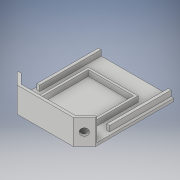
# Autodesk Inventor part: bottom-housing
Saved by Autodesk Inventor 2018 (Build 220112000, 112)
## iProperties
Created: 2019-10-14
Part Number: bottom-housing
Material: Generic
Document SubType Name: Modeling
Designer: jklei
Density: 1 g/cm^3
Appearance: Default
Author: jklei
Autodesk Inventor part; units mm, degrees
ref_plane "YZ Plane" through (0, 0, 0) normal (1, 0, 0) x (0, 1, 0)
ref_plane "XZ Plane" through (0, 0, 0) normal (0, 1, 0) x (-1, 0, 0)
ref_plane "XY Plane" through (0, 0, 0) normal (0, 0, 1) x (1, 0, 0)
sketch "Sketch1" plane through (0, 0, 0) normal (0, 1, 0) x (-1, 0, 0)
  line L0 (0, 0) -> (88.9, 0)
  line L1 (88.9, 0) -> (88.9, -101.6)
  line L2 (88.9, -101.6) -> (0, -101.6)
  line L3 (0, -101.6) -> (0, 0)
  dimension "d0" = 88.9
  dimension "d1" = 101.6
  constraints: 8 end point, 2 parallel, 1 horizontal, 1 perpendicular
  measures "d0" distance of L1.end L2.end
  measures "d1" distance of L0.end L1.end
extrude "Extrusion1" add sketch "Sketch1" along normal blind 3.175
chamfer "Chamfer1" distance 12.7 angle 45 2 edges at (-88.9, 1.5875, 0) (0, 1.5875, 0)
sketch "Sketch9" plane through (0, 3.175, 0) normal (0, 1, 0) x (1, 0, 0)
  line L0 (0, 12.7) -> (-12.7, 0) projected
  line L1 (0, 12.7) -> (0, 101.6) projected
  line L2 (0, 101.6) -> (-88.9, 101.6) projected
  line L3 (-88.9, 101.6) -> (-88.9, 12.7) projected
  line L4 (-76.2, 0) -> (-88.9, 12.7) projected
  line L5 (-76.2, 0) -> (-12.7, 0) projected
  line L6 (-3.175, 14.0151) -> (-14.0151, 3.175)
  line L7 (-14.0151, 3.175) -> (-74.8849, 3.175)
  line L8 (-74.8849, 3.175) -> (-85.725, 14.0151)
  line L9 (-88.9, 101.6) -> (0, 101.6) projected
  line L10 (-85.725, 14.0151) -> (-88.9, 14.0151)
  line L11 (-88.9, 12.7) -> (-88.9, 101.6) projected
  line L12 (-3.175, 14.0151) -> (0, 14.0151)
  point P0 (0, 0)
  point P1 (-3.175, 98.425)
  point P2 (-3.175, 101.6)
  dimension "d42" = 87.5849
  constraints: 10 end point, 3 point on line, 2 horizontal, 2 other
  measures "d42" distance between parallel lines of L2 L12
extrude "Extrusion8" add sketch "Sketch9" along normal blind 25.4 contours L0 L5 L4 L3 L10 L8 L7 L6 L12 L1
sketch "Sketch12" plane through (0, 3.175, 0) normal (0, 1, 0) x (1, 0, 0)
  line L0 (0, 101.6) -> (-88.9, 101.6) projected
  line L1 (0, 101.6) -> (-3.175, 101.6)
  line L2 (-14.0151, 3.175) -> (-3.175, 14.0151) projected
  line L3 (-3.175, 101.6) -> (-6.35, 101.6)
  line L4 (-6.35, 101.6) -> (-6.35, 31.75)
  line L5 (-6.35, 31.75) -> (-3.175, 31.75)
  line L6 (-3.175, 31.75) -> (-3.175, 101.6)
  line L7 (-88.9, 101.6) -> (-85.725, 101.6)
  line L8 (-85.725, 101.6) -> (-82.55, 101.6)
  line L9 (-82.55, 101.6) -> (-82.55, 31.75)
  line L10 (-82.55, 31.75) -> (-85.725, 31.75)
  line L11 (-85.725, 31.75) -> (-85.725, 101.6)
  point P0 (0, 0)
  dimension "d34" = 3.175
  dimension "d35" = 3.175
  dimension "d36" = 69.85
  dimension "d37" = 3.175
  dimension "d38" = 3.175
  dimension "d39" = 69.85
  constraints: 20 end point, 4 parallel, 2 horizontal, 2 perpendicular, 2 point on line
  measures "d34" distance of L0.start L1.end
  measures "d35" distance of L5.end L4.end
  measures "d36" distance of L4.end L3.end
  measures "d37" distance of L0.end L7.end
  measures "d38" distance of L9.end L10.end
  measures "d39" distance of L8.end L9.end
extrude "Extrusion10" add sketch "Sketch12" along normal blind 6.35
sketch "Sketch13" plane through (-12.7, 0, 0) normal (0.7071068, 0, 0.7071068) x (0.7071068, 0, -0.7071068)
  line L0 (0, 28.575) -> (0, 0) projected
  line L1 (0, 14.2875) -> (17.824, 14.2875)
  circle A0 centre (8.912, 14.2875) radius 4.15
  point P0 (8.9803, 0)
  dimension "d43" = 8.3
  constraints: 2 end point, 2 midpoint, 1 centre point, 1 horizontal
  measures "d43" diameter of A0
extrude "Extrusion11" cut sketch "Sketch13" against normal up to next
sketch "Sketch14" plane through (-88.9, 0, -12.7) normal (-0.7071068, 0, 0.7071068) x (0.7071068, 0, 0.7071068)
  line L0 (17.9605, 0) -> (17.9605, 28.575) projected
  line L1 (17.9605, 14.2875) -> (0, 14.2875)
  line L2 (0, 28.575) -> (0, 0) projected
  circle A0 centre (8.9803, 14.2875) radius 4.15
  point P0 (71.842, 0)
  dimension "d46" = 8.3
  constraints: 3 midpoint, 2 end point, 1 centre point
  measures "d46" diameter of A0
extrude "Extrusion12" cut sketch "Sketch14" against normal up to next
sketch "Sketch15" plane through (0, 3.175, 0) normal (0, 1, 0) x (1, 0, 0)
  line L0 (-69.85, 74.295) -> (-19.05, 74.295)
  line L1 (-19.05, 74.295) -> (-19.05, 9.525)
  line L2 (-19.05, 9.525) -> (-69.85, 9.525)
  line L3 (-69.85, 9.525) -> (-69.85, 74.295)
  line L4 (-6.35, 31.75) -> (-6.35, 101.6) projected
  line L5 (0, 14.0151) -> (0, 101.6) projected
  line L6 (-18.796, 74.549) -> (-70.104, 74.549)
  line L7 (-70.104, 74.549) -> (-70.104, 9.271)
  line L8 (-70.104, 9.271) -> (-18.796, 9.271)
  line L9 (-18.796, 9.271) -> (-18.796, 74.549)
  line L10 (-72.644, 77.089) -> (-16.256, 77.089)
  line L11 (-16.256, 77.089) -> (-16.256, 6.731)
  line L12 (-16.256, 6.731) -> (-72.644, 6.731)
  line L13 (-72.644, 6.731) -> (-72.644, 77.089)
  line L14 (-14.0151, 3.175) -> (-74.8849, 3.175) projected
  point P0 (0, 0)
  dimension "d49" = 50.8
  dimension "d50" = 64.77
  dimension "d52" = 19.05
  dimension "d53" = 0.254
  dimension "d54" = 2.54
  dimension "d57" = 6.35
  constraints: 24 end point, 6 parallel, 3 perpendicular, 1 horizontal, 6 other
  measures "d49" distance of L1.end L2.end
  measures "d50" distance of L0.end L1.end
  measures "d52" distance between parallel lines of L5 L1
  measures "d53" distance between parallel lines of L0 L6
  measures "d54" distance between parallel lines of L6 L10
  measures "d57" distance between parallel lines of L14 L2
extrude "Extrusion13" add sketch "Sketch15" along normal blind 6.35 contours L10 L11 L12 L13
body "Solid1"
